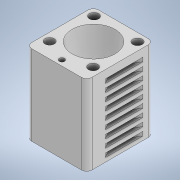
# Autodesk Inventor part: cylinder incomplete
Saved by Autodesk Inventor 2020 (Build 240168000, 168)
## iProperties
Created: 2020-08-04
Part Number: cylinder incomplete
Material: Generic
Document SubType Name: Modeling
Designer: benny
Density: 1 g/cm^3
Appearance: Default
Author: benny
Autodesk Inventor part; units mm, degrees
ref_plane "YZ Plane" through (0, 0, 0) normal (1, 0, 0) x (0, 1, 0)
ref_plane "XZ Plane" through (0, 0, 0) normal (0, 1, 0) x (-1, 0, 0)
ref_plane "XY Plane" through (0, 0, 0) normal (0, 0, 1) x (1, 0, 0)
sketch "Sketch1" plane through (0, 0, 0) normal (0, 1, 0) x (-1, 0, 0)
  line L0 (22.5, 25) -> (-22.5, 25)
  line L1 (-22.5, 25) -> (-22.5, -25)
  line L2 (-22.5, -25) -> (22.5, -25)
  line L3 (22.5, -25) -> (22.5, 25)
  line L4 (22.5, 25) -> (-22.5, -25) construction
  line L5 (-22.5, 25) -> (22.5, -25) construction
  point P0 (0, 0)
  dimension "d0" = 45
  dimension "d1" = 50
  constraints: 12 end point, 2 midpoint, 2 parallel, 1 horizontal, 1 perpendicular
  measures "d0" distance of L2.end L1.end
  measures "d1" distance of L1.end L0.end
extrude "Extrusion1" add sketch "Sketch1" along normal blind 60
fillet "Fillet1" radius 4 4 edges at (22.5, 30, 25) (-22.5, 30, 25) (22.5, 30, -25) (-22.5, 30, -25)
sketch "Sketch2" plane through (0, 60, 0) normal (0, 1, 0) x (1, 0, 0)
  circle A0 centre (0, 2.6667) radius 16
  point P0 (0, 0)
  dimension "d5" = 32
  constraints: 1 centre point
  measures "d5" diameter of A0
extrude "Extrusion2" cut sketch "Sketch2" against normal blind 60
ref_plane "Work Plane3" through (0, 3, 0) normal (0, -1, 0) x (1, 0, 0)
sketch "Sketch13" plane through (0, 3, 0) normal (0, -1, 0) x (1, 0, 0)
  circle A0 centre (42, -3) radius 24
  point P0 (0, 0)
  dimension "d27" = 48
  constraints: 1 centre point
  measures "d27" diameter of A0
extrude "Extrusion7" cut sketch "Sketch13" against normal blind 3
ref_plane "Work Plane4" through (0, 9, 0) normal (0, -1, 0) x (1, 0, 0)
sketch "Sketch14" plane through (0, 9, 0) normal (0, -1, 0) x (1, 0, 0)
  circle A0 centre (42, -3) radius 24
  point P0 (0, 0)
  dimension "d34" = 48
  constraints: 1 centre point
  measures "d34" diameter of A0
extrude "Extrusion8" cut sketch "Sketch14" against normal blind 3
ref_plane "Work Plane12" through (0, 15, 0) normal (0, -1, 0) x (1, 0, 0)
sketch "Sketch15" plane through (0, 15, 0) normal (0, -1, 0) x (1, 0, 0)
  circle A0 centre (42, -3) radius 24
  point P0 (0, 0)
  dimension "d41" = 48
  constraints: 1 centre point
  measures "d41" diameter of A0
extrude "Extrusion9" cut sketch "Sketch15" against normal blind 3
ref_plane "Work Plane13" through (0, 21, 0) normal (0, -1, 0) x (1, 0, 0)
sketch "Sketch16" plane through (0, 21, 0) normal (0, -1, 0) x (1, 0, 0)
  arc A0 (22.5, 10.9911) -> (22.5, -16.9911) centre (42, -3) ccw projected
  circle A1 centre (42, -3) radius 24
  point P0 (0, 0)
  point P1 (22.5, -16.9911)
  dimension "d45" = 48
  constraints: 1 centre point, 1 coincident
  measures "d45" diameter of A1
extrude "Extrusion10" cut sketch "Sketch16" against normal blind 3
ref_plane "Work Plane14" through (0, 27, 0) normal (0, -1, 0) x (1, 0, 0)
sketch "Sketch17" plane through (0, 27, 0) normal (0, -1, 0) x (1, 0, 0)
  circle A0 centre (42, -3) radius 24
  point P0 (0, 0)
  dimension "d49" = 48
  constraints: 1 centre point
  measures "d49" diameter of A0
extrude "Extrusion11" cut sketch "Sketch17" against normal blind 3
ref_plane "Work Plane15" through (0, 33, 0) normal (0, -1, 0) x (1, 0, 0)
sketch "Sketch18" plane through (0, 33, 0) normal (0, -1, 0) x (1, 0, 0)
  circle A0 centre (42, -3) radius 24
  point P0 (0, 0)
  dimension "d53" = 48
  constraints: 1 centre point
  measures "d53" diameter of A0
extrude "Extrusion12" cut sketch "Sketch18" against normal blind 3
ref_plane "Work Plane16" through (0, 39, 0) normal (0, -1, 0) x (1, 0, 0)
sketch "Sketch19" plane through (0, 39, 0) normal (0, -1, 0) x (1, 0, 0)
  circle A0 centre (42, -3) radius 24
  point P0 (0, 0)
  dimension "d57" = 48
  constraints: 1 centre point
  measures "d57" diameter of A0
extrude "Extrusion13" cut sketch "Sketch19" against normal blind 3
ref_plane "Work Plane17" through (0, 45, 0) normal (0, -1, 0) x (1, 0, 0)
sketch "Sketch20" plane through (0, 45, 0) normal (0, -1, 0) x (1, 0, 0)
  circle A0 centre (42, -3) radius 24
  point P0 (0, 0)
  dimension "d61" = 48
  constraints: 1 centre point
  measures "d61" diameter of A0
extrude "Extrusion14" cut sketch "Sketch20" against normal blind 3
ref_plane "Work Plane18" through (0, 51, 0) normal (0, -1, 0) x (1, 0, 0)
sketch "Sketch21" plane through (0, 51, 0) normal (0, -1, 0) x (1, 0, 0)
  circle A0 centre (42, -3) radius 24
  point P0 (0, 0)
  dimension "d65" = 48
  constraints: 1 centre point
  measures "d65" diameter of A0
extrude "Extrusion15" cut sketch "Sketch21" against normal blind 3
mirror "Mirror1" about plane through (0, 0, 0) normal (1, 0, 0) of "Extrusion7", "Extrusion8", "Extrusion9", "Extrusion10", "Extrusion11", "Extrusion12", "Extrusion13", "Extrusion14", "Extrusion15"
pattern_circular "Circular Pattern3" count 2 over 90 about axis through (0, 60, -2.6667) along (0, 1, 0) of "Extrusion15", "Extrusion14", "Extrusion13", "Extrusion12", "Extrusion11", "Extrusion10", "Extrusion9", "Extrusion8", "Extrusion7"
sketch "Sketch22" plane through (0, 0, 0) normal (0, -1, 0) x (1, 0, 0)
  line L0 (2, 11) -> (-2, 11)
  line L1 (-2, 11) -> (-2, 21)
  line L2 (-2, 21) -> (2, 21)
  line L3 (2, 21) -> (2, 11)
  line L4 (2, 11) -> (-2, 21) construction
  line L5 (-2, 11) -> (2, 21) construction
  point P0 (0, 0)
  point P1 (0, 16)
  dimension "d74" = 4
  dimension "d75" = 10
  constraints: 12 end point, 2 midpoint, 2 parallel, 1 horizontal, 1 perpendicular
  measures "d74" distance of L1.end L2.end
  measures "d75" distance of L0.end L1.end
extrude "Extrusion16" cut sketch "Sketch22" against normal blind 2
sketch "Sketch23" plane through (0, 0, 0) normal (0, -1, 0) x (1, 0, 0)
  line L0 (0, 0) -> (0, 21)
  line L1 (-2, 13.2078) -> (-2, 21) projected
  constraints: 2 end point, 1 parallel
sketch "Sketch24" plane through (0, 0, 0) normal (0, -1, 0) x (1, 0, 0)
  circle A0 centre (0, 21) radius 2
  point P0 (0, 0)
  dimension "d78" = 4
  constraints: 1 centre point
  measures "d78" diameter of A0
extrude "Extrusion17" cut sketch "Sketch24" against normal blind 62
sketch "Sketch25" plane through (0, 0, 21) normal (0, -1, 0) x (1, 0, 0)
  point P0 (0, -21)
sketch "Sketch27" plane through (0, 60, 0) normal (0, 1, 0) x (1, 0, 0)
  line L0 (0, 3) -> (-16.2635, 19.2635)
  line L1 (0, 3) -> (23, 3) construction
  circle A0 centre (-16.2635, 19.2635) radius 3.5
  point P0 (0, 0)
  dimension "d91" = 23
  dimension "d92" = 135
  dimension "d93" = 7
  constraints: 4 end point, 1 centre point, 1 coincident, 1 equal length, 1 horizontal
  measures "d91" distance of L0.start L0.end
  measures "d92" angle of L1 L0
  measures "d93" diameter of A0
extrude "Extrusion18" cut sketch "Sketch27" against normal blind 60
pattern_circular "Circular Pattern5" count 4 over 360 about axis through (0, 60, -2.6667) along (0, -1, 0) of "Extrusion18"
body "Solid1"
